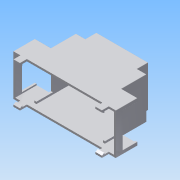
# Autodesk Inventor part: D2MG корпус
Saved by Autodesk Inventor 2015 SP1 (Build 190203100, 203)
## iProperties
Created: 2017-11-06
Part Number: D2MG корпус
Material: Типовые
Document SubType Name: Modeling
Designer: Влад
Density: 1 g/cm^3
Appearance: Белый пластик
Author: Влад
Autodesk Inventor part; units mm, degrees
sketch "Эскиз1" plane through (0, 0, 0) normal (0, 0, 1) x (1, 0, 0)
  line L0 (45.1, -6.35) -> (45.1, -25.35)
  line L1 (45.1, -25.35) -> (-45.1, -25.35)
  line L2 (-45.1, -25.35) -> (-45.1, -6.35)
  line L3 (-31, 15.65) -> (-31, -6.35)
  line L4 (31, 15.65) -> (31, -6.35)
  line L5 (-22.75, 25.35) -> (-22.75, 15.65)
  line L6 (22.75, 25.35) -> (22.75, 15.65)
  line L7 (-22.75, 25.35) -> (22.75, 25.35)
  line L8 (-45.1, -6.35) -> (-31, -6.35)
  line L9 (31, -6.35) -> (45.1, -6.35)
  line L10 (-31, 15.65) -> (-22.75, 15.65)
  line L11 (22.75, 15.65) -> (31, 15.65)
  line L12 (45.1, -25.35) -> (-45.1, 25.35) construction
  line L13 (-45.1, -25.35) -> (45.1, 25.35) construction
  point P0 (0, 0)
  point P1 (0, 0)
  dimension "d0" = 90.2
  dimension "d5" = 22.35
  dimension "d8" = 22.35
  dimension "d12" = 14.1
  dimension "d13" = 14.1
  dimension "d14" = 62
  dimension "d15" = 45.5
  dimension "d16" = 50.7
  dimension "d17" = 19
  dimension "d18" = 41
  constraints: 28 end point, 5 horizontal, 4 vertical, 2 parallel, 1 coincident, 1 midpoint, 1 perpendicular
  measures "d0" distance of L0.end L1.end
  measures "d5" distance between parallel lines of L0 L6
  measures "d8" distance between parallel lines of L2 L5
  measures "d12" distance between parallel lines of L0 L4
  measures "d13" distance between parallel lines of L2 L3
  measures "d14" distance between parallel lines of L4 L3
  measures "d15" distance between parallel lines of L6 L5
  measures "d16" distance between parallel lines of L1 L7
  measures "d17" distance between parallel lines of L1 L9
  measures "d18" distance between parallel lines of L1 L11
extrude "Выдавливание1" add sketch "Эскиз1" along normal blind 1.75
ref_plane "РабПлоскость1" through (0, 0, 36.3) normal (0, 0, 1) x (1, 0, 0)
sketch "Эскиз2" plane through (0, 0, 36.3) normal (0, 0, 1) x (1, 0, 0)
  line L0 (-45.1, -6.35) -> (-45.1, -25.35) projected
  line L1 (-45.1, -25.35) -> (45.1, -25.35) projected
  line L2 (45.1, -25.35) -> (45.1, -6.35) projected
  line L3 (45.1, -6.35) -> (31, -6.35) projected
  line L4 (31, -6.35) -> (31, 15.65) projected
  line L5 (31, 15.65) -> (22.75, 15.65) projected
  line L6 (22.75, 15.65) -> (22.75, 25.35) projected
  line L7 (22.75, 25.35) -> (-22.75, 25.35) projected
  line L8 (-22.75, 25.35) -> (-22.75, 15.65) projected
  line L9 (-22.75, 15.65) -> (-31, 15.65) projected
  line L10 (-31, 15.65) -> (-31, -6.35) projected
  line L11 (-31, -6.35) -> (-45.1, -6.35) projected
  point P0 (0, 0)
extrude "Выдавливание2" add sketch "Эскиз2" against normal blind 1.75
sketch "Эскиз3" plane through (45.1, -25.35, 0) normal (1, 0, 0) x (0, 0, -1)
  line L0 (-1.75, 19) -> (-1.75, 0)
  line L1 (-1.75, 0) -> (-34.55, 0)
  line L2 (-34.55, 0) -> (-34.55, 19)
  line L3 (-33.3, 19) -> (-33.3, 6)
  line L4 (-3, 19) -> (-3, 6)
  line L5 (-33.3, 6) -> (-3, 6)
  line L6 (-36.3, 0) -> (-36.3, 19) projected
  line L7 (0, 0) -> (0, 19) projected
  line L8 (-34.55, 19) -> (-33.3, 19)
  line L9 (-3, 19) -> (-1.75, 19)
  point P0 (0, 25.35)
  dimension "d26" = 6
  dimension "d27" = 3
  dimension "d28" = 3
  constraints: 16 end point, 4 perpendicular, 3 horizontal, 3 parallel
  measures "d26" distance between parallel lines of L1 L5
  measures "d27" distance between parallel lines of L6 L3
  measures "d28" distance between parallel lines of L7 L4
extrude "Выдавливание3" add sketch "Эскиз3" against normal blind 1.7
sketch "Эскиз4" plane through (31, -6.35, 0) normal (1, 0, 0) x (0, 0, -1)
  line L0 (-34.55, 22) -> (-1.75, 22)
  line L1 (-1.75, 22) -> (-1.75, 0)
  line L2 (-1.75, 0) -> (-34.55, 0)
  line L3 (-34.55, 0) -> (-34.55, 22)
  point P0 (0, 6.35)
  constraints: 8 end point, 2 parallel, 1 horizontal, 1 perpendicular
extrude "Выдавливание4" add sketch "Эскиз4" against normal blind 1.8
sketch "Эскиз5" plane through (22.75, 15.65, 0) normal (1, 0, 0) x (0, 0, -1)
  line L0 (-34.55, 9.7) -> (-1.75, 9.7)
  line L1 (-1.75, 9.7) -> (-1.75, 0)
  line L2 (-1.75, 0) -> (-34.55, 0)
  line L3 (-34.55, 0) -> (-34.55, 9.7)
  point P0 (0, -15.65)
  constraints: 8 end point, 2 parallel, 1 horizontal, 1 perpendicular
extrude "Выдавливание5" add sketch "Эскиз5" against normal blind 1.8
sketch "Эскиз6" plane through (22.75, 15.65, 0) normal (0, 1, 0) x (1, 0, 0)
  line L0 (0, -34.55) -> (6.45, -34.55)
  line L1 (6.45, -1.75) -> (0, -1.75)
  line L2 (0, -1.75) -> (0, -34.55)
  line L3 (4.45, -15.15) -> (6.45, -15.15)
  line L4 (6.45, -21.15) -> (4.45, -21.15)
  line L5 (4.45, -21.15) -> (4.45, -15.15)
  line L6 (6.45, -34.55) -> (6.45, -21.15)
  line L7 (6.45, -15.15) -> (6.45, -1.75)
  point P0 (-22.75, 0)
  dimension "d37" = 13.4
  dimension "d38" = 6
  dimension "d39" = 2
  constraints: 16 end point, 4 parallel, 2 horizontal, 2 perpendicular
  measures "d37" distance between parallel lines of L0 L4
  measures "d38" distance of L4.end L3.start
  measures "d39" distance of L3.start L3.end
extrude "Выдавливание6" add sketch "Эскиз6" against normal blind 1.8
sketch "Эскиз7" plane through (31, -6.35, 0) normal (1, 0, 0) x (0, 0, -1)
  line L0 (-34.55, -19) -> (-34.55, 0) projected
  line L1 (-34.55, 0) -> (-34.55, -14.5)
  line L2 (-1.75, -14.5) -> (-1.75, 0)
  line L3 (-32.75, 0) -> (-32.75, -14.5)
  line L4 (-3.55, 0) -> (-3.55, -14.5)
  line L5 (-1.75, 0) -> (-3.55, 0)
  line L6 (-32.75, 0) -> (-34.55, 0)
  line L7 (-34.55, -14.5) -> (-32.75, -14.5)
  line L8 (-3.55, -14.5) -> (-1.75, -14.5)
  point P0 (0, 6.35)
  dimension "d42" = 14.5
  dimension "d43" = 1.8
  dimension "d44" = 1.8
  constraints: 16 end point, 5 parallel, 2 horizontal, 2 perpendicular, 2 vertical, 1 point on line
  measures "d42" distance of L1.end L1.start
  measures "d43" distance between parallel lines of L0 L3
  measures "d44" distance between parallel lines of L4 L2
extrude "Выдавливание7" add sketch "Эскиз7" against normal blind 1.8
mirror "Зеркальное отражение2" about plane through (0, 0, 0) normal (1, 0, 0) of "Выдавливание3", "Выдавливание4", "Выдавливание5", "Выдавливание6", "Выдавливание7"
sketch "Эскиз8" plane through (-22.75, 25.35, 0) normal (0, 1, 0) x (1, 0, 0)
  line L0 (43.7, -34.55) -> (43.7, -1.75) projected
  line L1 (1.8, -1.75) -> (43.7, -1.75)
  line L2 (43.7, -1.75) -> (43.7, -2)
  line L3 (43.7, -2) -> (1.8, -2)
  line L4 (1.8, -2) -> (1.8, -1.75)
  line L5 (1.8, -34.55) -> (43.7, -34.55)
  line L6 (43.7, -34.55) -> (43.7, -34.3)
  line L7 (43.7, -34.3) -> (1.8, -34.3)
  line L8 (1.8, -34.3) -> (1.8, -34.55)
  point P0 (22.75, 0)
  dimension "d47" = 0.25
  dimension "d48" = 0.25
  constraints: 16 end point, 4 parallel, 2 horizontal, 2 perpendicular, 2 point on line
  measures "d47" distance between parallel lines of L3 L1
  measures "d48" distance between parallel lines of L7 L5
extrude "Выдавливание8" add sketch "Эскиз8" against normal blind 2.5
ref_plane "РабПлоскость2" through (-22.75, 22.85, 0) normal (0, 1, 0) x (1, 0, 0)
sketch "Эскиз9" plane through (-22.75, 22.85, 0) normal (0, 1, 0) x (1, 0, 0)
  line L0 (1.8, -1.75) -> (43.7, -1.75)
  line L1 (43.7, -34.55) -> (1.8, -34.55)
  line L2 (25.85, -32.15) -> (25.85, -33.9)
  line L3 (19.65, -33.9) -> (19.65, -32.15)
  line L4 (25.85, -2.4) -> (25.85, -4.15)
  line L5 (19.65, -4.15) -> (19.65, -2.4)
  line L6 (1.8, -15.15) -> (3.5, -15.15)
  line L7 (3.5, -21.15) -> (1.8, -21.15)
  line L8 (42, -15.15) -> (43.7, -15.15)
  line L9 (43.7, -21.15) -> (42, -21.15)
  line L10 (19.65, -2.4) -> (25.85, -2.4)
  line L11 (19.65, -33.9) -> (25.85, -33.9)
  line L12 (3.5, -32.15) -> (19.65, -32.15)
  line L13 (25.85, -32.15) -> (42, -32.15)
  line L14 (3.5, -4.15) -> (19.65, -4.15)
  line L15 (25.85, -4.15) -> (42, -4.15)
  line L16 (3.5, -4.15) -> (3.5, -15.15)
  line L17 (3.5, -21.15) -> (3.5, -32.15)
  line L18 (42, -4.15) -> (42, -15.15)
  line L19 (42, -21.15) -> (42, -32.15)
  line L20 (1.8, -34.55) -> (1.8, -21.15)
  line L21 (1.8, -15.15) -> (1.8, -1.75)
  line L22 (43.7, -1.75) -> (43.7, -15.15)
  line L23 (43.7, -21.15) -> (43.7, -34.55)
  dimension "d58" = 6.2
  dimension "d59" = 6.2
  dimension "d62" = 6
  dimension "d63" = 6
  constraints: 48 end point, 10 perpendicular, 9 parallel, 6 vertical, 5 horizontal
  measures "d58" distance between parallel lines of L2 L3
  measures "d59" distance between parallel lines of L4 L5
  measures "d62" distance between parallel lines of L9 L8
  measures "d63" distance between parallel lines of L7 L6
extrude "Выдавливание9" add sketch "Эскиз9" against normal blind 1.75
sketch "Эскиз10" plane through (-22.75, 22.85, 0) normal (0, 1, 0) x (1, 0, 0)
  circle A0 centre (3.5, -4.15) radius 1.75
  circle A1 centre (42, -4.15) radius 1.75
  circle A2 centre (42, -32.15) radius 1.75
  circle A3 centre (3.5, -32.15) radius 1.75
  point P0 (22.75, 0)
  dimension "d76" = 3.5
  dimension "d77" = 3.5
  dimension "d78" = 3.5
  dimension "d79" = 3.5
  constraints: 4 centre point
  measures "d76" diameter of A0
  measures "d77" diameter of A1
  measures "d78" diameter of A2
  measures "d79" diameter of A3
extrude "Выдавливание10" add sketch "Эскиз10" against normal blind 5.5
sketch "Эскиз11" plane through (-22.75, 22.85, 0) normal (0, 1, 0) x (1, 0, 0)
  circle A0 centre (3.5, -4.15) radius 1
  circle A1 centre (42, -4.15) radius 1
  arc A2 (40.25, -32.15) -> (43.7, -32.5653) centre (42, -32.15) ccw projected
  circle A3 centre (42, -32.15) radius 1
  circle A4 centre (3.5, -32.15) radius 1
  point P0 (22.75, 0)
  dimension "d82" = 2
  dimension "d83" = 2
  dimension "d84" = 2
  dimension "d85" = 2
  constraints: 4 centre point, 1 coincident
  measures "d82" diameter of A0
  measures "d83" diameter of A1
  measures "d84" diameter of A3
  measures "d85" diameter of A4
extrude "Выдавливание11" cut sketch "Эскиз11" against normal blind 4
fillet "Сопряжение1" radius 0.3 26 edges at (0, 25.35, 36.3) (22.75, 20.5, 36.3) (26.875, 15.65, 36.3) (31, 15.65, 18.15) (22.75, 25.35, 18.15) (31, 4.65, 36.3) (38.05, -6.35, 36.3) (45.1, -15.85, 36.3) (-22.75, 20.5, 36.3) (-26.875, 15.65, 36.3) (-31, 4.65, 36.3) (-31, 15.65, 18.15) (-38.05, -6.35, 36.3) (-45.1, -15.85, 36.3) (0, 25.35, 0) (22.75, 20.5, 0) (26.875, 15.65, 0) (31, 4.65, 0) (38.05, -6.35, 0) (45.1, -15.85, 0) (-22.75, 20.5, 0) (-26.875, 15.65, 0) (-22.75, 25.35, 18.15) (-31, 4.65, 0) (-38.05, -6.35, 0) (-45.1, -15.85, 0)
fillet "Сопряжение2" radius 0.1 8 edges at (28.2, 15.65, 21.15) (29.2, 15.65, 18.15) (28.2, 15.65, 15.15) (27.2, 15.65, 18.15) (-28.2, 15.65, 21.15) (-27.2, 15.65, 18.15) (-29.2, 15.65, 18.15) (-28.2, 15.65, 15.15)
fillet "Сопряжение3" radius 0.2 10 edges at (-45.1, -12.85, 33.3) (-44.25, -6.35, 33.3) (-45.1, -19.35, 18.15) (-44.25, -6.35, 3) (-45.1, -12.85, 3) (44.25, -6.35, 33.3) (45.1, -12.85, 33.3) (45.1, -19.35, 18.15) (44.25, -6.35, 3) (45.1, -12.85, 3)
fillet "Сопряжение4" radius 0.3 12 edges at (45.0414, -6.4086, 2.9414) (45.0121, -6.4379, 0.0879) (45.1, -6.35, 1.55) (45.0414, -6.4086, 33.3586) (45.0121, -6.4379, 36.2121) (45.1, -6.35, 34.75) (-45.0414, -6.4086, 33.3586) (-45.0121, -6.4379, 36.2121) (-45.1, -6.35, 34.75) (-45.0414, -6.4086, 2.9414) (-45.0121, -6.4379, 0.0879) (-45.1, -6.35, 1.55)
sketch "Эскиз12" plane through (0, 0, 36.3) normal (0, 0, 1) x (1, 0, 0)
  line L0 (33.1, -25.35) -> (38.9, -25.35)
  line L1 (38.9, -25.35) -> (38.9, -31.35)
  line L2 (38.9, -31.35) -> (33.1, -31.35)
  line L3 (33.1, -31.35) -> (33.1, -25.35)
  line L4 (-44.8, -25.35) -> (44.8, -25.35) projected
  line L5 (45.1, -25.35) -> (45.1, -6.65) projected
  line L6 (-38.9, -25.35) -> (-33.1, -25.35)
  line L7 (-33.1, -25.35) -> (-33.1, -31.35)
  line L8 (-33.1, -31.35) -> (-38.9, -31.35)
  line L9 (-38.9, -31.35) -> (-38.9, -25.35)
  line L10 (-45.1, -6.65) -> (-45.1, -25.35) projected
  point P0 (0, 0)
  point P1 (36, -25.35)
  point P2 (-36, -25.35)
  dimension "d92" = 5.8
  dimension "d93" = 6
  dimension "d94" = 6.2
  dimension "d95" = 5.8
  dimension "d96" = 6
  dimension "d97" = 6.2
  constraints: 16 end point, 4 parallel, 2 horizontal, 2 midpoint, 2 perpendicular, 2 point on line
  measures "d92" distance of L1.end L2.end
  measures "d93" distance of L0.end L1.end
  measures "d94" distance between parallel lines of L5 L1
  measures "d95" distance of L7.end L8.end
  measures "d96" distance of L6.end L7.end
  measures "d97" distance between parallel lines of L10 L9
extrude "Выдавливание12" add sketch "Эскиз12" against normal blind 1.75
sketch "Эскиз13" plane through (38.9, -31.35, 36.3) normal (1, 0, 0) x (0, 0, -1)
  line L0 (3, 2) -> (1.75, 2)
  line L1 (1.75, 2) -> (1.75, 0)
  line L2 (3, 2) -> (1.75, 0)
  point P0 (36.3, 31.35)
  dimension "d104" = 1.25
  dimension "d105" = 2
  constraints: 6 end point
  measures "d104" distance of L0.start L0.end
  measures "d105" distance of L0.end L1.end
extrude "Выдавливание13" add sketch "Эскиз13" against normal blind 5.8
sketch "Эскиз14" plane through (-38.9, -31.35, 36.3) normal (-1, 0, 0) x (0, 0, 1)
  line L0 (-1.75, 0) -> (-3, 2)
  line L1 (-3, 2) -> (-1.75, 0) projected
  line L2 (-3, 2) -> (-1.75, 2)
  line L3 (-1.75, 2) -> (-3, 2) projected
  line L4 (-1.75, 2) -> (-1.75, 0)
  line L5 (-1.75, 6) -> (-1.75, 0) projected
  point P0 (-36.3, 31.35)
  constraints: 6 end point, 3 collinear
extrude "Выдавливание14" add sketch "Эскиз14" against normal blind 5.8
ref_plane "РабПлоскость3" through (0, 0, 18.15) normal (0, 0, 1) x (1, 0, 0)
mirror "Зеркальное отражение3" about plane through (0, 0, 18.15) normal (0, 0, 1) of "Выдавливание12", "Выдавливание13", "Выдавливание14"
fillet "Сопряжение5" radius 0.2 12 edges at (33.1, -28.35, 0) (38.9, -28.35, 0) (36, -31.35, 0) (-38.9, -28.35, 0) (-36, -31.35, 0) (-33.1, -28.35, 0) (-38.9, -28.35, 36.3) (-36, -31.35, 36.3) (-33.1, -28.35, 36.3) (33.1, -28.35, 36.3) (36, -31.35, 36.3) (38.9, -28.35, 36.3)
